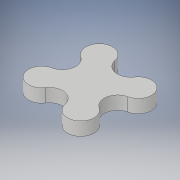
# Autodesk Inventor part: Turret Drive Gear
Saved by Autodesk Inventor 2019.4 (Build 234330000, 330)
## iProperties
Created: 2020-01-29
Part Number: Turret Drive Gear
Material: Generic
Document SubType Name: Modeling
Designer: admin
Density: 1 g/cm^3
Appearance: Default
Author: admin
Autodesk Inventor part; units mm, degrees
ref_plane "YZ Plane" through (0, 0, 0) normal (1, 0, 0) x (0, 1, 0)
ref_plane "XZ Plane" through (0, 0, 0) normal (0, 1, 0) x (-1, 0, 0)
ref_plane "XY Plane" through (0, 0, 0) normal (0, 0, 1) x (1, 0, 0)
sketch "Sketch1" plane through (0, 0, 0) normal (0, 1, 0) x (-1, 0, 0)
  circle A0 centre (0, 0) radius 13.0656 construction
  arc A1 (11.8215, 2.442) -> (13.4456, 11.5876) centre (10.81, 7.3386) ccw
  arc A2 (11.8215, 2.442) -> (10.0858, -6.6323) centre (12.833, -2.4547) ccw
  arc A3 (2.442, -11.8215) -> (10.0858, -6.6323) centre (7.3386, -10.81) ccw
  arc A4 (2.442, -11.8215) -> (-6.6323, -10.0858) centre (-2.4547, -12.833) ccw
  arc A5 (-11.2725, -12.3171) -> (-6.6323, -10.0858) centre (-10.81, -7.3386) ccw
  line L0 (7.922, -1.5153) -> (0, 0)
  line L1 (0, 0) -> (-1.5153, -7.922)
  dimension "d0" = 5
  dimension "d1" = 5
  dimension "d2" = 5
  dimension "d3" = 5
  dimension "d4" = 5
  dimension "d5" = 90
  constraints: 17 point on circle, 6 centre point, 4 end point, 4 equal radius, 1 coincident
  measures "d0" radius of A1
  measures "d1" radius of A2
  measures "d2" radius of A3
  measures "d3" radius of A4
  measures "d4" radius of A5
  measures "d5" angle of L1 L0
extrude "Extrusion1" add sketch "Sketch1" along normal blind 5
pattern_circular "Circular Pattern1" count 4 over 360 about axis through (0, 0, 0) along (0, 1, 0) of "Extrusion1"
equation "\"d1\" = d0"
equation "\"d2\" = d0"
equation "\"d3\" = d0"
equation "\"d4\" = d0"
body "Solid1"
